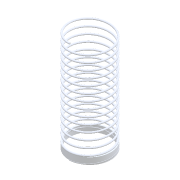
# Autodesk Inventor part: 00_Spring_15mm_6mm
Saved by Autodesk Inventor 2022 (Build 260153000, 153)
## iProperties
Created: 2022-07-31
Part Number: 00_Spring_15mm_6mm
Material: Generisch
Document SubType Name: Modeling
Designer: diederichbenedict
Density: 1 g/cm^3
Appearance: Vorgabe
Author: diederichbenedict
Autodesk Inventor part; units mm, degrees
ref_plane "YZ Plane" through (0, 0, 0) normal (1, 0, 0) x (0, 1, 0)
ref_plane "XZ Plane" through (0, 0, 0) normal (0, 1, 0) x (-1, 0, 0)
ref_plane "XY Plane" through (0, 0, 0) normal (0, 0, 1) x (1, 0, 0)
sketch "Skizze1" plane through (0, 0, 0) normal (1, 0, 0) x (0, 1, 0)
  circle A0 centre (0, 3) radius 0.125
  point P0 (0, 0)
  dimension "d0" = 0.25
  dimension "d1" = 3
  constraints: 1 centre point
  measures "d0" diameter of A0
  measures "d1" distance of point (0, 0) A0.centre
coil "Spirale1" sketch "Skizze1" operation add axis through (0, -10, 0) along (0, 1, 0) pitch 1 turns 15 hand right
sketch "Skizze2" plane through (0, 0, 0) normal (0, 1, 0) x (-1, 0, 0)
  line L0 (0, 2.875) -> (0, 3.125) projected
  line L1 (0, 3.125) -> (0, 2.875) projected
  circle A0 centre (0, 0) radius 2.914
  circle A1 centre (0, 0) radius 3.105
  point P0 (0, 3)
  point P1 (0, 3)
  constraints: 2 centre point, 2 coincident
extrude "Extrusion1" add sketch "Skizze2" along normal blind 1
